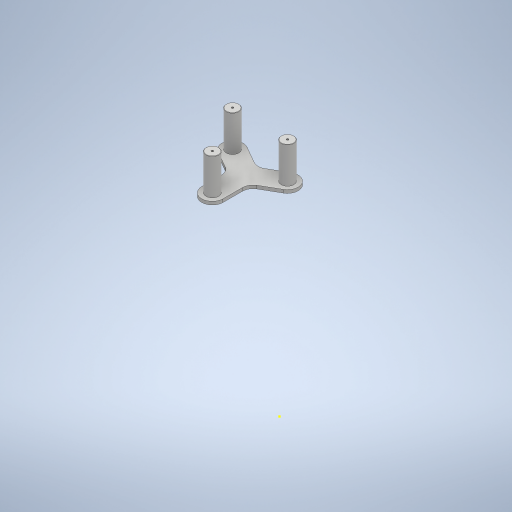
# Autodesk Inventor part: 零件1
Saved by Autodesk Inventor 2023 (Build 270158000, 158)
## iProperties
Created: 2023-04-30
Part Number: 零件1
Material: 常规
Document SubType Name: Sheet Metal
Designer: 47376
Density: 1 g/cm^3
Sheet Metal Rule: Default_mm
Appearance: 默认
Author: 47376
Autodesk Inventor part; units mm, degrees
ref_plane "YZ Plane" through (0, 0, 0) normal (1, 0, 0) x (0, 1, 0)
ref_plane "XZ Plane" through (0, 0, 0) normal (0, 1, 0) x (-1, 0, 0)
ref_plane "XY Plane" through (0, 0, 0) normal (0, 0, 1) x (1, 0, 0)
ref_plane "工作平面5" through (-8, 0, 4.5) normal (0, 0, 1) x (1, 0, 0)
sketch "草图5" plane through (-8, 0, 4.5) normal (0, 0, 1) x (1, 0, 0)
  arc A0 (-229.373, 177.0271) -> (-229.1311, 177.052) centre (-230.6821, 190.9658) ccw
  circle A1 centre (-229.4321, 193.1309) radius 6
  circle A2 centre (-177.5679, 193.1309) radius 6
  circle A3 centre (-203.5, 148.2151) radius 6
  arc A4 (-172.5679, 184.4706) -> (-182.5679, 201.7911) centre (-177.5679, 193.1309) ccw
  arc A5 (-224.4321, 201.7911) -> (-234.4321, 184.4706) centre (-229.4321, 193.1309) ccw
  arc A6 (-213.5, 148.2151) -> (-193.5, 148.2151) centre (-203.5, 148.2151) ccw
  line L0 (-234.4321, 184.4706) -> (-218.5, 175.2722)
  line L1 (-172.5679, 184.4706) -> (-188.5, 175.2722)
  line L2 (-224.4321, 201.7911) -> (-208.5, 192.5927)
  line L3 (-182.5679, 201.7911) -> (-198.5, 192.5927)
  line L4 (-213.5, 148.2151) -> (-213.5, 166.6119)
  line L5 (-193.5, 148.2151) -> (-193.5, 166.6119)
  line L6 (-206, 177.7999) -> (-206, 178.2297)
  arc A7 (-208.5, 192.5927) -> (-198.5, 192.5927) centre (-203.5, 201.2529) ccw
  arc A8 (-188.5, 175.2722) -> (-193.5, 166.6119) centre (-183.5, 166.6119) ccw
  arc A9 (-213.5, 166.6119) -> (-218.5, 175.2722) centre (-223.5, 166.6119) ccw
  point P0 (8, 0)
  point P1 (-184.4262, 177.6242)
  point P2 (-222.5767, 177.6259)
  dimension "d31" = 12
  dimension "d33" = 12
  dimension "d37" = 20
  dimension "d38" = 20
  dimension "d44" = 10
  dimension "d87" = 12
  constraints: 14 end point, 14 point on circle, 10 centre point, 10 tangent, 2 coincident, 2 equal radius, 2 point on line, 1 vertical
  measures "d31" diameter of A1
  measures "d33" diameter of A3
  measures "d37" diameter of A5
  measures "d38" diameter of A6
  measures "d44" radius of A7
  measures "d87" diameter of A2
extrude "拉伸1" add sketch "草图5" along normal blind 3
ref_plane "工作平面2" through (-8, 0, 7.5) normal (0, 0, 1) x (1, 0, 0)
sketch "草图8" plane through (-8, 0, 4.5) normal (0, 0, -1) x (-1, 0, 0)
  circle A0 centre (203.5, 148.2151) radius 6 projected
  circle A1 centre (203.5, 148.2151) radius 6
  circle A2 centre (229.4321, 193.1309) radius 6 projected
  circle A3 centre (229.4321, 193.1309) radius 6
  circle A4 centre (177.5679, 193.1309) radius 6 projected
  circle A5 centre (177.5679, 193.1309) radius 6
  point P0 (-8, 0)
  constraints: 3 centre point, 3 coincident
sketch "草图9" plane through (-8, 0, 4.5) normal (0, 0, -1) x (-1, 0, 0)
  point P0 (-8, 0)
extrude "拉伸3" add sketch "草图8" against normal blind 37
hole "孔4" at (-237.4321, 193.1309, 41.5) direction (0, 0, -1) diameter 1.941 depth 10 tip angle 118 thread size "3-48 UNC" class "2B" standard "ANSI Unified Screw Threads"
hole "孔5" at (-185.5679, 193.1309, 41.5) direction (0, 0, -1) diameter 1.941 depth 10 tip angle 118 thread size "3-48 UNC" class "2B" standard "ANSI Unified Screw Threads"
hole "孔6" at (-211.5, 148.2151, 41.5) direction (0, 0, -1) diameter 1.941 depth 10 tip angle 118 thread size "3-48 UNC" class "2B" standard "ANSI Unified Screw Threads"
fillet "圆角4" radius 0.3 3 edges at (-231.4321, 193.1309, 41.5) (-179.5679, 193.1309, 41.5) (-205.5, 148.2151, 41.5)
sketch "草图10" plane through (-8, 0, 4.5) normal (0, 0, -1) x (-1, 0, 0)
  circle A0 centre (229.4321, 193.1309) radius 6
  circle A1 centre (203.5, 148.2151) radius 6
  circle A2 centre (177.5679, 193.1309) radius 6.4097
  point P0 (-8, 0)
  constraints: 3 centre point, 3 coincident
extrude "拉伸4" cut sketch "草图10" against normal blind 1
equation "\"折弯半径\" = 厚度"
equation "\"折弯释压宽度\" = 厚度"
equation "\"折弯释压深度\" = 0.5 * 厚度"
equation "\"拐角释压尺寸\" = 4 * 厚度"
equation "\"最小余量\" = 2 * 厚度"
equation "\"过渡半径\" = 折弯半径"
equation "\"Jacobi半径尺寸\" = 折弯半径"
equation "\"间隙大小\" = 厚度"
equation "\"厚度\" = 0.5"
